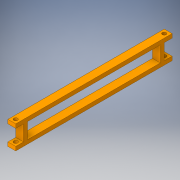
# Autodesk Inventor part: arm
Saved by Autodesk Inventor 2016 (Build 200138000, 138)
## iProperties
Created: 2018-01-19
Part Number: arm
Material: Generic
Document SubType Name: Modeling
Designer: New User
Density: 1 g/cm^3
Appearance: Default
Author: New User
Autodesk Inventor part; units mm, degrees
ref_plane "YZ Plane" through (0, 0, 0) normal (1, 0, 0) x (0, 1, 0)
ref_plane "XZ Plane" through (0, 0, 0) normal (0, 1, 0) x (-1, 0, 0)
ref_plane "XY Plane" through (0, 0, 0) normal (0, 0, 1) x (1, 0, 0)
sketch "Sketch1" plane through (0, 0, 0) normal (0, 1, 0) x (-1, 0, 0)
  line L0 (0, 0) -> (-50.8, 0)
  line L1 (-50.8, 0) -> (-50.8, -1016)
  line L2 (-50.8, -1016) -> (0, -1016)
  line L3 (0, -1016) -> (0, 0)
  dimension "d0" = 1016
  dimension "d1" = 50.8
  constraints: 8 end point, 2 parallel, 1 horizontal, 1 perpendicular
  measures "d0" distance of L2.end L0.start
  measures "d1" distance of L0.start L0.end
extrude "Extrusion1" add sketch "Sketch1" along normal blind 25.4
sketch "Sketch2" plane through (0, 25.4, 0) normal (0, 1, 0) x (1, 0, 0)
  line L0 (0, 50.8) -> (50.8, 50.8)
  line L1 (50.8, 50.8) -> (50.8, 76.2)
  line L2 (50.8, 76.2) -> (0, 76.2)
  line L3 (0, 76.2) -> (0, 50.8)
  line L4 (0, 965.2) -> (50.8, 965.2)
  line L5 (50.8, 965.2) -> (50.8, 939.8)
  line L6 (50.8, 939.8) -> (0, 939.8)
  line L7 (0, 939.8) -> (0, 965.2)
  line L8 (50.8, 1016) -> (0, 1016) projected
  line L9 (0, 0) -> (50.8, 0) projected
  dimension "d5" = 25.4
  dimension "d12" = 25.4
  dimension "d16" = 50.8
  dimension "d17" = 50.8
  constraints: 16 end point, 4 parallel, 2 horizontal, 2 perpendicular
  measures "d5" distance between parallel lines of L2 L0
  measures "d12" distance between parallel lines of L4 L6
  measures "d16" distance between parallel lines of L8 L4
  measures "d17" distance between parallel lines of L9 L0
extrude "Extrusion2" add sketch "Sketch2" along normal blind 101.6
sketch "Sketch3" plane through (0, 25.4, 0) normal (0, 1, 0) x (1, 0, 0)
  circle A0 centre (25.4, 25.4) radius 12.7
  line L0 (0, 50.8) -> (0, 0) projected
  line L1 (0, 0) -> (50.8, 0) projected
  circle A1 centre (25.4, 990.6) radius 12.7
  line L2 (50.8, 1016) -> (0, 1016) projected
  line L3 (50.8, 965.2) -> (50.8, 1016) projected
  dimension "d18" = 25.4
  dimension "d19" = 25.4
  dimension "d20" = 25.4
  dimension "d21" = 25.4
  dimension "d22" = 25.4
  dimension "d23" = 25.4
  constraints: 2 centre point
  measures "d18" diameter of A0
  measures "d19" distance from line of A0.centre L0
  measures "d20" distance from line of L1 A0.centre
  measures "d21" diameter of A1
  measures "d22" distance from line of L2 A1.centre
  measures "d23" distance from line of L3 A1.centre
sketch "Sketch4" plane through (0, 127, 0) normal (0, 1, 0) x (1, 0, 0)
  line L0 (0, 0) -> (50.8, 0)
  line L1 (50.8, 0) -> (50.8, 1016)
  line L2 (50.8, 1016) -> (0, 1016)
  line L3 (0, 1016) -> (0, 0)
  constraints: 8 end point, 2 parallel, 1 horizontal, 1 perpendicular
extrude "Extrusion3" add sketch "Sketch4" along normal blind 25.4
extrude "Extrusion4" cut sketch "Sketch3" along normal blind 174.625 and the other way blind 63.5
body "Solid1"
